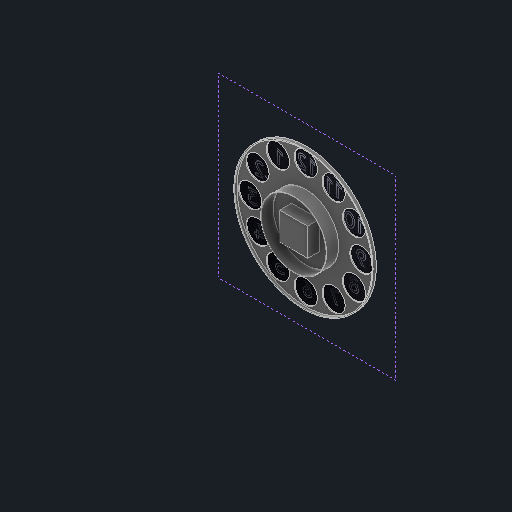
# Autodesk Inventor part: Clock
Saved by Autodesk Inventor 2023.1 (Build 271208000, 208)
## iProperties
Created: 2023-08-24
Part Number: Clock
Material: Generic
Document SubType Name: Modeling
Designer: washichi
Density: 1 g/cm^3
Appearance: Fine Textured - Black
Author: washichi
Autodesk Inventor part; units mm, degrees
ref_plane "YZ Plane" through (0, 0, 0) normal (1, 0, 0) x (0, 1, 0)
ref_plane "XZ Plane" through (0, 0, 0) normal (0, 1, 0) x (-1, 0, 0)
ref_plane "XY Plane" through (0, 0, 0) normal (0, 0, 1) x (1, 0, 0)
sketch "Sketch1" plane through (0, 0, 0) normal (0, 0, 1) x (1, 0, 0)
  circle A0 centre (0, 0) radius 150
  circle A1 centre (0, 120) radius 25
  circle A2 centre (60, 103.923) radius 25
  circle A3 centre (103.923, 60) radius 25
  circle A4 centre (120, 0) radius 25
  circle A5 centre (103.923, -60) radius 25
  circle A6 centre (60, -103.923) radius 25
  circle A7 centre (0, -120) radius 25
  circle A8 centre (-60, -103.923) radius 25
  circle A9 centre (-103.923, -60) radius 25
  circle A10 centre (-120, 0) radius 25
  circle A11 centre (-103.923, 60) radius 25
  circle A12 centre (-60, 103.923) radius 25
  dimension "d0" = 300
  dimension "d1" = 50
  dimension "d2" = 0
  dimension "d3" = 120
  dimension "d6" = 360
  constraints: 13 centre point, 1 coincident, 37 other
  measures "d0" diameter of A0
  measures "d1" diameter of A1
  measures "d2" horizontal distance of point (0, 0) A1.centre
  measures "d3" distance of point (0, 0) A1.centre
extrude "Extrusion1" add sketch "Sketch1" along normal blind 2
sketch "Sketch2" plane through (0, 0, 2) normal (0, 0, 1) x (1, 0, 0)
  circle A0 centre (0, 0) radius 150 projected
  circle A1 centre (0, 0) radius 148
  dimension "d10" = 2
  constraints: 1 centre point
  measures "d10" radial gap between concentric circles of A0 A1
extrude "Extrusion2" add sketch "Sketch2" along normal blind 5
sketch "Sketch3" plane through (0, 0, 2) normal (0, 0, 1) x (1, 0, 0)
  circle A0 centre (0, 0) radius 71
  circle A1 centre (0, 0) radius 70
  line L0 (30, 30) -> (-30, 30)
  line L1 (-30, 30) -> (-30, -30)
  line L2 (-30, -30) -> (30, -30)
  line L3 (30, -30) -> (30, 30)
  line L4 (30, 30) -> (-30, -30) construction
  line L5 (-30, 30) -> (30, -30) construction
  dimension "d13" = 142
  dimension "d14" = 1
  dimension "d17" = 60
  dimension "d18" = 60
  constraints: 12 end point, 2 centre point, 2 midpoint, 2 parallel, 1 coincident, 1 horizontal, 1 perpendicular
  measures "d13" diameter of A0
  measures "d14" radial gap between concentric circles of A0 A1
  measures "d17" distance of L2.end L1.end
  measures "d18" distance of L1.end L0.end
extrude "Extrusion3" add sketch "Sketch3" along normal blind 26
sketch "Sketch4" plane through (0, 0, 0) normal (0, 0, 1) x (1, 0, 0)
  point P0 (0, 0)
sketch "Sketch5" plane through (0, 0, 0) normal (0, 0, -1) x (-1, 0, 0)
  line L0 (-191.5583, 191.5583) -> (190.3872, 191.5583) construction
  line L1 (190.3872, 191.5583) -> (190.3872, -190.3872) construction
  line L2 (190.3872, -190.3872) -> (-191.5583, -190.3872) construction
  line L3 (-191.5583, -190.3872) -> (-191.5583, 191.5583) construction
  point P0 (0, 0)
  constraints: 2 other
body "Solid1"
